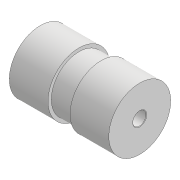
# Autodesk Inventor part: Вал конвейера
Saved by Autodesk Inventor 2022 (Build 260153000, 153)
## iProperties
Created: 2023-02-18
Part Number: Вал конвейера
Material: Типовые
Document SubType Name: Modeling
Designer: Глеб
Density: 1 g/cm^3
Appearance: По умолчанию
Author: Глеб
Autodesk Inventor part; units mm, degrees
ref_plane "YZ Plane" through (0, 0, 0) normal (1, 0, 0) x (0, 1, 0)
ref_plane "XZ Plane" through (0, 0, 0) normal (0, 1, 0) x (-1, 0, 0)
ref_plane "XY Plane" through (0, 0, 0) normal (0, 0, 1) x (1, 0, 0)
sketch "Эскиз1" plane through (0, 0, 0) normal (1, 0, 0) x (0, 1, 0)
  circle A0 centre (0, 0) radius 14
  dimension "d0" = 28
  constraints: 1 centre point, 1 coincident
  measures "d0" diameter of A0
extrude "Выдавливание1" add sketch "Эскиз1" along normal mid plane 45
sketch "Эскиз2" plane through (22.5, 0, 0) normal (1, 0, 0) x (0, 0, -1)
  point P0 (0, 0)
  point P1 (0, 0)
  constraints: 1 coincident
hole "Отверстие1" at (22.5, 0, 0) direction (-1, 0, 0) diameter 6 depth 60
fillet "Сопряжение1" radius 0.2 2 edges at (22.5, 0, 3) (-22.5, 0, 3)
ref_plane "РабПлоскость2" through (-14.5, 2.1629, 84.9725) normal (-1, 0, 0) x (0, -0.9996762, 0.0254464)
sketch "Эскиз4" plane through (-14.5, 2.1629, 84.9725) normal (-1, 0, 0) x (0, -0.9996762, 0.0254464)
  circle A0 centre (0, -85) radius 10
  circle A1 centre (0, -85) radius 3.2 projected
  circle A2 centre (0, -85) radius 14
  dimension "d14" = 20
  constraints: 2 centre point, 2 coincident
  measures "d14" diameter of A0
extrude "Выдавливание3" cut sketch "Эскиз4" against normal blind 12 contours A2
